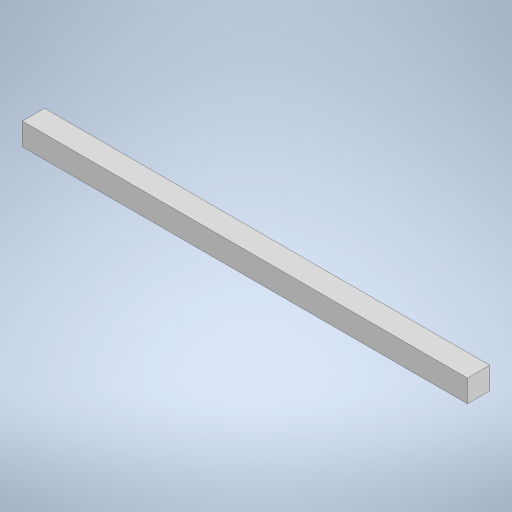
# Autodesk Inventor part: przewód
Saved by Autodesk Inventor 2023 (Build 270158000, 158)
## iProperties
Created: 2024-02-01
Part Number: przewód
Material: Ogólny
Document SubType Name: Modeling
Designer: domin
Density: 1 g/cm^3
Appearance: Domyślna
Author: domin
Autodesk Inventor part; units mm, degrees
ref_plane "YZ Plane" through (0, 0, 0) normal (1, 0, 0) x (0, 1, 0)
ref_plane "XZ Plane" through (0, 0, 0) normal (0, 1, 0) x (-1, 0, 0)
ref_plane "XY Plane" through (0, 0, 0) normal (0, 0, 1) x (1, 0, 0)
sketch "Szkic1" plane through (0, 0, 0) normal (0, 0, 1) x (1, 0, 0)
  line L0 (0, 0) -> (0, 1)
  line L1 (0, 1) -> (20, 1)
  line L2 (20, 1) -> (20, 0)
  line L3 (20, 0) -> (0, 0)
  dimension "d0" = 1
  dimension "d1" = 20
  constraints: 8 end point, 3 perpendicular, 1 vertical
  measures "d0" distance of L0.start L0.end
  measures "d1" distance of L0.end L1.end
extrude "Wyciągnięcie proste1" add sketch "Szkic1" along normal blind 1
